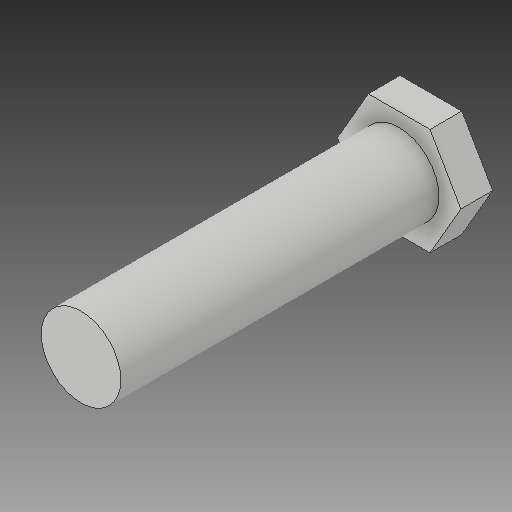
# Autodesk Inventor part: Tornillo
Saved by Autodesk Inventor 2019 (Build 230136000, 136)
## iProperties
Created: 2019-07-02
Part Number: Tornillo
Material: Generic
Document SubType Name: Modeling
Designer: Oscar Rojas
Density: 1 g/cm^3
Appearance: Default
Mass: 3.76761 g
Surface Area: 17.5592 cm^2
Volume: 3.76761 cm^3
Author: Oscar Rojas
Autodesk Inventor part; units mm, degrees
ref_plane "YZ Plane" through (0, 0, 0) normal (1, 0, 0) x (0, 1, 0)
ref_plane "XZ Plane" through (0, 0, 0) normal (0, 1, 0) x (-1, 0, 0)
ref_plane "XY Plane" through (0, 0, 0) normal (0, 0, 1) x (1, 0, 0)
sketch "Sketch1" plane through (0, 0, 0) normal (0, 0, 1) x (1, 0, 0)
  circle A0 centre (0, 0) radius 5
  dimension "d0" = 10
  constraints: 1 centre point, 1 coincident
  measures "d0" diameter of A0
extrude "Extrusion1" add sketch "Sketch1" along normal blind 40
sketch "Sketch2" plane through (0, 0, 0) normal (0, 0, -1) x (-1, 0, 0)
  line L0 (-7.7614, 0) -> (-3.8807, 6.7215)
  line L1 (-3.8807, 6.7215) -> (3.8807, 6.7215)
  line L2 (3.8807, 6.7215) -> (7.7614, 0)
  line L3 (7.7614, 0) -> (3.8807, -6.7215)
  line L4 (3.8807, -6.7215) -> (-3.8807, -6.7215)
  line L5 (-3.8807, -6.7215) -> (-7.7614, 0)
  point P0 (0, 0)
  point P1 (0, 0)
  constraints: 12 end point, 1 coincident, 13 other
extrude "Extrusion2" add sketch "Sketch2" along normal blind 4
body "Solid1"
